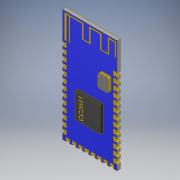
# Autodesk Inventor part: HM-10
Saved by Autodesk Inventor 2019.3 (Build 233278000, 278)
## iProperties
Created: 2019-03-19
Part Number: HM-10
Material: Типовые
Document SubType Name: Modeling
Designer: Boris
Density: 1 g/cm^3
Appearance: Металл — 2400F
Author: Boris
Autodesk Inventor part; units mm, degrees
ref_plane "РабПлоскость2" through (0, 0, 0.01) normal (0, 0, 1) x (1, 0, 0)
sketch "Эскиз1" plane through (0, 0, 0.01) normal (0, 0, 1) x (1, 0, 0)
  line L0 (-0.45, 7.1) -> (12.55, 7.1)
  line L1 (12.55, 7.1) -> (12.55, -19.8)
  line L2 (12.55, -19.8) -> (-0.45, -19.8)
  line L3 (-0.45, -19.8) -> (-0.45, 7.1)
  point P0 (0, 0)
  point P1 (-0.45, 0)
  dimension "d1" = 13
  dimension "d2" = 26.9
  dimension "d3" = 7.1
  dimension "d4" = 0.45
  constraints: 8 end point, 2 parallel, 1 horizontal, 1 perpendicular, 1 point on line
  measures "d1" distance of L0.start L0.end
  measures "d2" distance of L0.end L1.end
  measures "d3" distance from line of point (0, 0) L0
  measures "d4" distance from line of L3 point (0, 0)
extrude "Выдавливание1" add sketch "Эскиз1" along normal blind 0.8
sketch "Эскиз2" plane through (0, 0, 0.81) normal (0, 0, 1) x (1, 0, 0)
  line L0 (0.45, 0.5) -> (-0.45, 0.5)
  line L1 (-0.45, 0.5) -> (-0.45, -0.5)
  line L2 (-0.45, -0.5) -> (0.45, -0.5)
  line L3 (0.45, -0.5) -> (0.45, 0.5)
  line L4 (0.45, 0.5) -> (-0.45, -0.5) construction
  line L5 (-0.45, 0.5) -> (0.45, -0.5) construction
  line L6 (-0.45, 7.1) -> (-0.45, -19.8) projected
  line L7 (12.55, 7.1) -> (-0.45, 7.1) projected
  point P0 (0, 0)
  point P1 (0, 0)
  point P2 (-0.45, 0)
  point P3 (0.45, 0)
  dimension "d7" = 0.9
  dimension "d8" = 1
  dimension "d9" = 7.1
  constraints: 12 end point, 3 midpoint, 2 parallel, 2 point on line, 1 horizontal, 1 horizontal alignment, 1 perpendicular
  measures "d7" distance of L2.end L1.end
  measures "d8" distance of L1.end L0.end
  measures "d9" distance from line of L7 point (0, 0)
ref_plane "РабПлоскость1" through (0, 0, 0.41) normal (0, 0, 1) x (1, 0, 0)
extrude "Выдавливание2" add sketch "Эскиз2" along normal blind 0.01
mirror "Зеркальное отражение1" about plane through (0, 0, 0.41) normal (0, 0, 1) of "Выдавливание2"
hole "Отверстие1" at (-0.45, 0, 0.81) direction (0, 0, -1) diameter 0.8 end through all both
pattern_linear "Прямоуг.массив1" count 13 spacing 1.5 along (0, -1, 0) of "Отверстие1", "Выдавливание2", "Зеркальное отражение1"
ref_plane "РабПлоскость3" through (6.05, 7.1, 0.01) normal (-1, 0, 0) x (0, 0, 1)
mirror "Зеркальное отражение2" about plane through (6.05, 7.1, 0.01) normal (-1, 0, 0) of "Отверстие1", "Выдавливание2", "Зеркальное отражение1", "Прямоуг.массив1"
sketch "Эскиз3" plane through (0, 0, 0.81) normal (0, 0, 1) x (1, 0, 0)
  line L0 (0.3, -18.9) -> (1.3, -18.9)
  line L1 (1.3, -18.9) -> (1.3, -19.8)
  line L2 (1.3, -19.8) -> (0.3, -19.8)
  line L3 (0.3, -19.8) -> (0.3, -18.9)
  line L4 (0.3, -18.9) -> (1.3, -19.8) construction
  line L5 (1.3, -18.9) -> (0.3, -19.8) construction
  line L6 (-0.45, -19.8) -> (12.55, -19.8) projected
  arc A0 (-0.45, -18.4) -> (-0.45, -17.6) centre (-0.45, -18) ccw projected
  line L7 (-0.45, -18.5) -> (-0.45, -19.8) projected
  line L8 (12.55, -19.8) -> (-0.45, -19.8) projected
  point P0 (0, 0)
  point P1 (0.8, -19.35)
  point P2 (0.8, -19.8)
  point P3 (0.8, -18.9)
  dimension "d23" = 1
  dimension "d24" = 0.9
  dimension "d25" = 1.8
  dimension "d26" = 1.25
  constraints: 12 end point, 3 midpoint, 2 parallel, 2 point on line, 1 horizontal, 1 perpendicular, 1 vertical alignment
  measures "d23" distance of L1.end L2.end
  measures "d24" distance of L0.end L1.end
  measures "d25" distance from line of L6 A0.centre
  measures "d26" distance from line of L7 point (0.8, -19.35)
extrude "Выдавливание3" add sketch "Эскиз3" along normal blind 0.01
mirror "Зеркальное отражение3" about plane through (0, 0, 0.41) normal (0, 0, 1) of "Выдавливание3"
hole "Отверстие2" at (0.8, -19.8, 0.81) direction (0, 0, -1) diameter 0.8 end through all both
pattern_linear "Прямоуг.массив2" count 8 spacing 1.5 along (1, 0, 0) of "Выдавливание3", "Зеркальное отражение3", "Отверстие2"
sketch "Эскиз4" plane through (0, 0, 0.81) normal (0, 0, 1) x (1, 0, 0)
  line L0 (0, 0.961) -> (0, 6.7155)
  line L1 (0, 6.7155) -> (4.5155, 6.7155)
  line L2 (4.5155, 6.7155) -> (4.5155, 3.4048)
  line L3 (4.5155, 3.4048) -> (5.908, 3.4048)
  line L4 (5.908, 3.4048) -> (5.908, 6.7155)
  line L5 (5.908, 6.7155) -> (8.8065, 6.7155)
  line L6 (8.8065, 6.7155) -> (8.8065, 3.4048)
  line L7 (8.8065, 3.4048) -> (10.3553, 3.4048)
  line L8 (10.3553, 3.4048) -> (10.3553, 6.7155)
  line L9 (10.3553, 6.7155) -> (12.2308, 6.7155)
  line L10 (12.2308, 6.7155) -> (12.2308, 3.4048)
  line L11 (12.2308, 3.4048) -> (12.0035, 3.4048)
  line L12 (12.0035, 3.4048) -> (12.0035, 6.4455)
  line L13 (12.0035, 6.4455) -> (10.611, 6.4455)
  line L14 (10.611, 6.4455) -> (10.611, 3.1775)
  line L15 (10.611, 3.1775) -> (8.494, 3.1775)
  line L16 (8.494, 3.1775) -> (8.494, 6.4455)
  line L17 (8.494, 6.4455) -> (6.2206, 6.4455)
  line L18 (6.2206, 6.4455) -> (6.2206, 3.1775)
  line L19 (6.2206, 3.1775) -> (4.2172, 3.1775)
  line L20 (4.2172, 3.1775) -> (4.2172, 6.4455)
  line L21 (4.2172, 6.4455) -> (1.3044, 6.4455)
  line L22 (1.3044, 6.4455) -> (1.3044, 0.961)
  line L23 (1.3044, 0.961) -> (1.0202, 0.961)
  line L24 (1.0202, 0.961) -> (1.0202, 6.4455)
  line L25 (1.0202, 6.4455) -> (0.4945, 6.4455)
  line L26 (0.4945, 6.4455) -> (0.4945, 0.961)
  line L27 (0.4945, 0.961) -> (0, 0.961)
  point P0 (0, 0)
  constraints: 56 end point, 18 perpendicular, 17 point on line, 1 parallel, 1 vertical
extrude "Выдавливание4" add sketch "Эскиз4" along normal blind 0.01
sketch "Эскиз5" plane through (0, 0, 0.81) normal (0, 0, 1) x (1, 0, 0)
  line L0 (3.25, -7.5) -> (9.25, -7.5)
  line L1 (9.25, -7.5) -> (9.25, -13.5)
  line L2 (9.25, -13.5) -> (3.25, -13.5)
  line L3 (3.25, -13.5) -> (3.25, -7.5)
  line L4 (3.25, -7.5) -> (9.25, -13.5) construction
  line L5 (9.25, -7.5) -> (3.25, -13.5) construction
  line L6 (12.55, -11.5) -> (12.55, -11) projected
  line L7 (8.8, -19.8) -> (9.3, -19.8) projected
  point P0 (0, 0)
  point P1 (6.25, -10.5)
  dimension "d41" = 6
  dimension "d42" = 6
  dimension "d43" = 3.3
  dimension "d44" = 6.3
  constraints: 12 end point, 2 midpoint, 2 parallel, 1 horizontal, 1 perpendicular
  measures "d41" distance of L1.end L2.end
  measures "d42" distance of L0.end L1.end
  measures "d43" distance between parallel lines of L6 L1
  measures "d44" distance between parallel lines of L7 L2
extrude "Выдавливание5" add sketch "Эскиз5" along normal blind 0.75
sketch "Эскиз6" plane through (0, 0, 0.81) normal (0, 0, 1) x (1, 0, 0)
  line L0 (8.65, -1) -> (11.15, -1)
  line L1 (11.15, -1) -> (11.15, -4.2)
  line L2 (11.15, -4.2) -> (8.65, -4.2)
  line L3 (8.65, -4.2) -> (8.65, -1)
  line L4 (8.65, -1) -> (11.15, -4.2) construction
  line L5 (11.15, -1) -> (8.65, -4.2) construction
  line L6 (-0.45, -2) -> (-0.45, -2.5) projected
  line L7 (12.55, 7.1) -> (-0.45, 7.1) projected
  point P0 (0, 0)
  point P1 (9.9, -2.6)
  dimension "d47" = 3.2
  dimension "d48" = 2.5
  dimension "d49" = 11.6
  dimension "d50" = 11.3
  constraints: 12 end point, 2 midpoint, 2 parallel, 1 horizontal, 1 perpendicular
  measures "d47" distance of L2.end L0.start
  measures "d48" distance of L0.start L0.end
  measures "d49" distance between parallel lines of L6 L1
  measures "d50" distance between parallel lines of L7 L2
extrude "Выдавливание6" add sketch "Эскиз6" along normal blind 0.75
fillet "Сопряжение1" radius 0.4 4 edges at (11.15, -4.2, 1.185) (8.65, -4.2, 1.185) (11.15, -1, 1.185) (8.65, -1, 1.185)
sketch "Эскиз7" plane through (0, 0, 1.56) normal (0, 0, 1) x (1, 0, 0)
  line L0 (4.1818, -13.025) -> (4.1818, 3.4839) construction
  line L1 (4.1818, 3.4839) -> (7.2246, 3.4839) construction
  line L2 (7.2246, 3.4839) -> (7.2246, -13.025) construction
  line L3 (7.2246, -13.025) -> (4.1818, -13.025) construction
  line L4 (4.848, -12.2041) -> (4.8815, -12.0715)
  spline S0 degree 2 poles (4.8815, -12.0715) (5.0446, -12.1134) (5.2161, -12.3291) (5.2161, -12.4854) knots 0 0 0 1 2 2 2
  spline S1 degree 2 poles (5.2161, -12.4854) (5.2161, -12.6469) (5.0843, -12.8497) (4.835, -12.9556) (4.6917, -12.9556) knots 0 0 0 1 2 3 3 3
  spline S2 degree 2 poles (4.6917, -12.9556) (4.5355, -12.9556) (4.3022, -12.836) (4.1818, -12.6157) (4.1818, -12.4831) knots 0 0 0 1 2 3 3 3
  spline S3 degree 2 poles (4.1818, -12.4831) (4.1818, -12.3329) (4.335, -12.1287) (4.473, -12.0883) knots 0 0 0 1 2 2 2
  line L5 (4.473, -12.0883) -> (4.5042, -12.2186)
  spline S4 degree 2 poles (4.5042, -12.2186) (4.3952, -12.2537) (4.2954, -12.3855) (4.2954, -12.4861) knots 0 0 0 1 2 2 2
  spline S5 degree 2 poles (4.2954, -12.4861) (4.2954, -12.6012) (4.4059, -12.7567) (4.5919, -12.8192) (4.691, -12.8192) knots 0 0 0 1 2 3 3 3
  spline S6 degree 2 poles (4.691, -12.8192) (4.8182, -12.8192) (5.0088, -12.7445) (5.1025, -12.5883) (5.1025, -12.4968) knots 0 0 0 1 2 3 3 3
  spline S7 degree 2 poles (5.1025, -12.4968) (5.1025, -12.3855) (4.9745, -12.2315) (4.848, -12.2041) knots 0 0 0 1 2 2 2
  line L6 (4.848, -11.195) -> (4.8815, -11.0623)
  spline S8 degree 2 poles (4.8815, -11.0623) (5.0446, -11.1043) (5.2161, -11.32) (5.2161, -11.4762) knots 0 0 0 1 2 2 2
  spline S9 degree 2 poles (5.2161, -11.4762) (5.2161, -11.6378) (5.0843, -11.8405) (4.835, -11.9465) (4.6917, -11.9465) knots 0 0 0 1 2 3 3 3
  spline S10 degree 2 poles (4.6917, -11.9465) (4.5355, -11.9465) (4.3022, -11.8268) (4.1818, -11.6065) (4.1818, -11.4739) knots 0 0 0 1 2 3 3 3
  spline S11 degree 2 poles (4.1818, -11.4739) (4.1818, -11.3238) (4.335, -11.1195) (4.473, -11.0791) knots 0 0 0 1 2 2 2
  line L7 (4.473, -11.0791) -> (4.5042, -11.2094)
  spline S12 degree 2 poles (4.5042, -11.2094) (4.3952, -11.2445) (4.2954, -11.3764) (4.2954, -11.477) knots 0 0 0 1 2 2 2
  spline S13 degree 2 poles (4.2954, -11.477) (4.2954, -11.5921) (4.4059, -11.7476) (4.5919, -11.8101) (4.691, -11.8101) knots 0 0 0 1 2 3 3 3
  spline S14 degree 2 poles (4.691, -11.8101) (4.8182, -11.8101) (5.0088, -11.7354) (5.1025, -11.5791) (5.1025, -11.4876) knots 0 0 0 1 2 3 3 3
  spline S15 degree 2 poles (5.1025, -11.4876) (5.1025, -11.3764) (4.9745, -11.2224) (4.848, -11.195) knots 0 0 0 1 2 2 2
  line L8 (5.0812, -10.304) -> (5.1993, -10.304)
  line L9 (5.1993, -10.304) -> (5.1993, -10.9648)
  spline S16 degree 2 poles (5.1993, -10.9648) (5.1551, -10.9663) (5.114, -10.9503) knots 0 0 0 1 1 1
  spline S17 degree 2 poles (5.114, -10.9503) (5.0461, -10.9251) (4.9158, -10.8139) (4.8297, -10.7087) knots 0 0 0 1 2 2 2
  spline S18 degree 2 poles (4.8297, -10.7087) (4.6955, -10.5463) (4.54, -10.432) (4.4699, -10.432) knots 0 0 0 1 2 2 2
  spline S19 degree 2 poles (4.4699, -10.432) (4.3968, -10.432) (4.2969, -10.5364) (4.2969, -10.6203) knots 0 0 0 1 2 2 2
  spline S20 degree 2 poles (4.2969, -10.6203) (4.2969, -10.7087) (4.4036, -10.8146) (4.4974, -10.8154) knots 0 0 0 1 2 2 2
  line L10 (4.4974, -10.8154) -> (4.4844, -10.9419)
  spline S21 degree 2 poles (4.4844, -10.9419) (4.3434, -10.929) (4.1955, -10.7598) (4.1955, -10.6172) knots 0 0 0 1 2 2 2
  spline S22 degree 2 poles (4.1955, -10.6172) (4.1955, -10.4732) (4.3548, -10.3055) (4.473, -10.3055) knots 0 0 0 1 2 2 2
  spline S23 degree 2 poles (4.473, -10.3055) (4.5332, -10.3055) (4.649, -10.3543) (4.7771, -10.4686) (4.8891, -10.6005) knots 0 0 0 1 2 3 3 3
  spline S24 degree 2 poles (4.8891, -10.6005) (4.9814, -10.711) (5.0477, -10.7735) (5.0812, -10.794) knots 0 0 0 1 2 2 2
  line L11 (5.0812, -10.794) -> (5.0812, -10.304)
  line L12 (4.9371, -10.1721) -> (4.9265, -10.0433)
  spline S25 degree 2 poles (4.9265, -10.0433) (5.021, -10.0288) (5.1155, -9.9251) (5.1155, -9.8512) knots 0 0 0 1 2 2 2
  spline S26 degree 2 poles (5.1155, -9.8512) (5.1155, -9.7613) (4.9814, -9.6393) (4.8708, -9.6393) knots 0 0 0 1 2 2 2
  spline S27 degree 2 poles (4.8708, -9.6393) (4.7657, -9.6393) (4.6437, -9.7567) (4.6437, -9.8527) knots 0 0 0 1 2 2 2
  spline S28 degree 2 poles (4.6437, -9.8527) (4.6437, -9.9122) (4.6978, -10.0075) (4.7413, -10.0349) knots 0 0 0 1 2 2 2
  line L13 (4.7413, -10.0349) -> (4.726, -10.15)
  line L14 (4.726, -10.15) -> (4.2123, -10.0532)
  line L15 (4.2123, -10.0532) -> (4.2123, -9.5562)
  line L16 (4.2123, -9.5562) -> (4.3297, -9.5562)
  line L17 (4.3297, -9.5562) -> (4.3297, -9.9549)
  line L18 (4.3297, -9.9549) -> (4.598, -10.009)
  spline S29 degree 2 poles (4.598, -10.009) (4.5355, -9.919) (4.5355, -9.82) knots 0 0 0 1 1 1
  spline S30 degree 2 poles (4.5355, -9.82) (4.5355, -9.6889) (4.7169, -9.509) (4.8594, -9.509) knots 0 0 0 1 2 2 2
  spline S31 degree 2 poles (4.8594, -9.509) (4.9958, -9.509) (5.0949, -9.5883) knots 0 0 0 1 1 1
  spline S32 degree 2 poles (5.0949, -9.5883) (5.2161, -9.6843) (5.2161, -9.8505) knots 0 0 0 1 1 1
  spline S33 degree 2 poles (5.2161, -9.8505) (5.2161, -9.9869) (5.0637, -10.1599) (4.9371, -10.1721) knots 0 0 0 1 2 2 2
  line L19 (5.1993, -9.0021) -> (4.96, -9.0021)
  line L20 (4.96, -9.0021) -> (4.96, -9.4358)
  line L21 (4.96, -9.4358) -> (4.8472, -9.4358)
  line L22 (4.8472, -9.4358) -> (4.1993, -8.98)
  line L23 (4.1993, -8.98) -> (4.1993, -8.8794)
  line L24 (4.1993, -8.8794) -> (4.8472, -8.8794)
  line L25 (4.8472, -8.8794) -> (4.8472, -8.7445)
  line L26 (4.8472, -8.7445) -> (4.96, -8.7445)
  line L27 (4.96, -8.7445) -> (4.96, -8.8794)
  line L28 (4.96, -8.8794) -> (5.1993, -8.8794)
  line L29 (5.1993, -8.8794) -> (5.1993, -9.0021)
  line L30 (4.8472, -9.0021) -> (4.396, -9.0021)
  line L31 (4.396, -9.0021) -> (4.8472, -9.3154)
  line L32 (4.8472, -9.3154) -> (4.8472, -9.0021)
  line L33 (5.1993, -8.1569) -> (5.1993, -8.2796)
  line L34 (5.1993, -8.2796) -> (4.4173, -8.2796)
  spline S34 degree 2 poles (4.4173, -8.2796) (4.4593, -8.3238) (4.5439, -8.4678) (4.5652, -8.525) knots 0 0 0 1 2 2 2
  line L35 (4.5652, -8.525) -> (4.4463, -8.525)
  spline S35 degree 2 poles (4.4463, -8.525) (4.3983, -8.4221) (4.2603, -8.2681) (4.1955, -8.2361) knots 0 0 0 1 2 2 2
  line L36 (4.1955, -8.2361) -> (4.1955, -8.1569)
  line L37 (4.1955, -8.1569) -> (5.1993, -8.1569)
  point P0 (0, 0)
  constraints: 1 vertical, 2 other
extrude "Выдавливание7" cut sketch "Эскиз7" against normal blind 0.01
